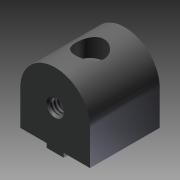
# Autodesk Inventor part: 4188_n
Saved by Autodesk Inventor 2016 (Build 200138000, 138)
## iProperties
Category: PARTsolutions
Company: 8020
Created: 2016-04-17
Part Number: 4188_n
Catalog Web Link: www.cadenas.de
Description: 4188, 4388_n-90 deg Pivot Nub
Vendor: 8020
Document SubType Name: Modeling
Designer: psAdmin
Manufacturer: 8020
Mass: 13.1896 g
Surface Area: 42.6466 cm^2
Volume: 13.1896 cm^3
Density: 1 g/cm^3
Material: Generic
Appearance: PSOLRGB-192-192-192
PSOL_IDENT_0: {$CADENAS_DATA\23d-libs\8020\inch\joining_plates\4188.prj},151 {VTYP=3D},{NB=4188_n},{LINA=4188_n},{
PSOL_IDENT_1: NN=4188, 4388_n},{DATE=22.08.2012},{GEOMDATE=05.01.2012 09:37:00},{VERSION=},{LINEID=10},{LINESUBID=
PSOL_IDENT_2: -1},{WBVAR=}  {NB=4188_n},{LINA=4188_n},{KT=DUMMY},{PN=4188},{A=1.000},{B=0.500},{C=1/4-20 SHCS},{D=
PSOL_IDENT_3: 1/4-20 Tap},{D1=0.2500},{W=.075},{CB=0.40600},{CBD=0.2750},{HD=0.25700},{X=0.060},{Y=0.245},{Z=0.250
PSOL_IDENT_4: },{TT=UNC},{BT=1/4-20},{BL=1.000},{NT=3382}
NN: 4188, 4388_n
NT: 3382
NB: 4188_n
NBSYN: $PN._n
LINA: 4188_n
PN: 4188
A: 1.000
B: 0.500
C: 1/4-20 SHCS
D: 1/4-20 Tap
D1: 0.2500
W: .075
CB: 0.40600
CBD: 0.2750
HD: 0.25700
X: 0.060
Y: 0.245
Z: 0.250
TT: UNC
BT: 1/4-20
BL: 1.000
SUPPLIER: 8020
ARTICLENO: 4188_n
BOMINFO: 4188_n
CREATOR: CADENAS GmbH
Title: 4188_n
Author: Cadenas PARTsolutions
Comments: 90 deg Pivot Nub
Autodesk Inventor part; units mm, degrees
ref_plane "YZ Plane" through (0, 0, 0) normal (1, 0, 0) x (0, 1, 0)
ref_plane "XZ Plane" through (0, 0, 0) normal (0, 1, 0) x (-1, 0, 0)
ref_plane "XY Plane" through (0, 0, 0) normal (0, 0, 1) x (1, 0, 0)
sketch "Sketch_1" plane through (0, 0, 0) normal (0, 0, 1) x (1, 0, 0)
  line L0 (-12.7, 0) -> (12.7, 0)
  line L1 (12.7, 0) -> (12.7, 12.7)
  arc A0 (12.7, 12.7) -> (-12.7, 12.7) centre (0, 12.7) ccw
  line L2 (-12.7, 12.7) -> (-12.7, 0)
  constraints: 6 end point, 2 point on circle, 1 centre point
extrude "Extrusion1" add sketch "Sketch_1" along normal mid plane 25.4
sketch "Sketch_7" plane through (0, 0, 12.7) normal (0, 0, 1) x (1, 0, 0)
  line L0 (-3.1115, -1.524) -> (3.1115, -1.524)
  line L1 (3.1115, -1.524) -> (3.1115, 0)
  line L2 (3.1115, 0) -> (-3.1115, 0)
  line L3 (-3.1115, 0) -> (-3.1115, -1.524)
  constraints: 8 end point
extrude "Extrusion2" add sketch "Sketch_7" against normal blind 6.35
sketch "Sketch_2" plane through (0, 0, -12.7) normal (0, 0, 1) x (1, 0, 0)
  line L0 (-3.1115, -1.524) -> (3.1115, -1.524)
  line L1 (3.1115, -1.524) -> (3.1115, 0)
  line L2 (3.1115, 0) -> (-3.1115, 0)
  line L3 (-3.1115, 0) -> (-3.1115, -1.524)
  constraints: 8 end point
extrude "Extrusion3" add sketch "Sketch_2" along normal blind 6.35
sketch "Sketch_3" plane through (0, 0, 0) normal (1, 0, 0) x (0, 1, 0)
  line L0 (12.7, -12.7) -> (12.7, 12.7)
  line L1 (12.7, 12.7) -> (15.875, 12.7)
  line L2 (15.875, 12.7) -> (15.1879, 12.0129)
  line L3 (15.1879, 12.0129) -> (15.1879, -12.0129)
  line L4 (15.1879, -12.0129) -> (15.875, -12.7)
  line L5 (15.875, -12.7) -> (12.7, -12.7)
  line L6 (12.7, -12.7) -> (12.7, 12.7)
  constraints: 14 end point
revolve "Revolution1" cut sketch "Sketch_3" angle 360 about axis through (0, 12.7, -12.7) along (0, 0, -1)
thread "Thread1" size "1/4-20 UNC" class "2B" standard "ANSI Unified Screw Threads" full length
sketch "Sketch_4" plane through (0, 0, 0) normal (0, 0, 1) x (1, 0, 0)
  line L0 (0, 0) -> (0, 25.4)
  line L1 (0, 25.4) -> (5.1562, 25.4)
  line L2 (5.1562, 25.4) -> (5.1562, 18.415)
  line L3 (5.1562, 18.415) -> (3.2639, 18.415)
  line L4 (3.2639, 18.415) -> (3.2639, 0)
  line L5 (3.2639, 0) -> (0, 0)
  line L6 (0, 0) -> (0, 25.4)
  constraints: 14 end point
revolve "Revolution2" cut sketch "Sketch_4" angle 360 about axis through (0, 0, 0) along (0, -1, 0)
ref_plane "nub_XY" through (0, 12.7, 12.7) normal (0, 0, 1) x (1, 0, 0)
ref_plane "nub_YZ" through (0, 12.7, 12.7) normal (1, 0, 0) x (0, 1, 0)
ref_plane "nub_ZX" through (0, 12.7, 12.7) normal (0, 1, 0) x (0, 0, 1)
ref_plane "nub1_XY" through (0, 12.7, -12.7) normal (0, 0, 1) x (1, 0, 0)
ref_plane "nub1_YZ" through (0, 12.7, -12.7) normal (1, 0, 0) x (0, 1, 0)
ref_plane "nub1_ZX" through (0, 12.7, -12.7) normal (0, 1, 0) x (0, 0, 1)
ref_plane "to_dummy_XY" through (0, 0, 0) normal (0, 1, 0) x (1, 0, 0)
ref_plane "to_dummy_YZ" through (0, 0, 0) normal (1, 0, 0) x (0, 0, -1)
ref_plane "to_dummy_ZX" through (0, 0, 0) normal (0, 0, -1) x (0, 1, 0)
ref_plane "to_screw_XY" through (0, 18.415, 0) normal (0, 1, 0) x (1, 0, 0)
ref_plane "to_screw_YZ" through (0, 18.415, 0) normal (1, 0, 0) x (0, 0, -1)
ref_plane "to_screw_ZX" through (0, 18.415, 0) normal (0, 0, -1) x (0, 1, 0)
body "Solid1"
